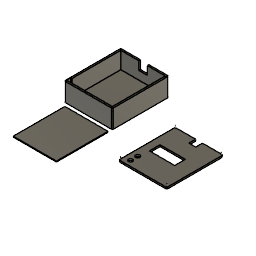
Case (Autodesk Fusion 360 design; units mm, degrees)
part number: 2025-12-30-11-50-45-676
Autodesk Fusion 360 part; units mm, degrees
sketch "Sketch1" plane through (0, 0, 0) normal (0, 0, 1) x (1, 0, 0)
  line L0 (0, 0) -> (53, 0)
  line L1 (53, 0) -> (53, -63)
  line L2 (53, -63) -> (0, -63)
  line L3 (0, -63) -> (0, 0)
  line L4 (-2, 2) -> (55, 2)
  line L5 (55, 2) -> (55, -65)
  line L6 (55, -65) -> (-2, -65)
  line L7 (-2, -65) -> (-2, 2)
  line L8 (0, -63) -> (-1.5, -63)
  line L9 (-1.5, -63) -> (-1.5, -58)
  line L10 (-1.5, -58) -> (0, -58)
  line L11 (0, -58) -> (0, -63)
  dimension "d1" = 53
  dimension "d2" = 63
  dimension "d7" = 1.5
  dimension "d8" = 5
  constraint horizontal L0
  constraint vertical L1
  constraint horizontal L2
  constraint vertical L3
  constraint coincident L0.start L3.end
  constraint horizontal L4
  constraint vertical L5
  constraint horizontal L6
  constraint vertical L7
  constraint horizontal L8
  constraint vertical L9
  constraint horizontal L10
  constraint vertical L11
  measures "d1" distance of L0.start L0.end
  measures "d2" distance of L0.start L2.end
  measures "d7" distance of L2.end L8.end
  measures "d8" distance of L2.end L10.end
extrude "Extrude1" add sketch "Sketch1" along normal blind 2 contours L0 L1 L2 L3 L11 | L3 L8 L9 L10 L11 makes body 1
extrude "Extrude2" add sketch "Sketch1" along normal blind 22 bodies 1
sketch "Sketch2" plane through (0, 0, 0) normal (0, 0, 1) x (1, 0, 0)
  line L0 (91.7333, -27) -> (148.7333, -27)
  line L1 (148.7333, -27) -> (148.7333, -94)
  line L2 (148.7333, -94) -> (91.7333, -94)
  line L3 (91.7333, -94) -> (91.7333, -27)
  line L4 (116.2333, -27) -> (124.2333, -27)
  line L5 (124.2333, -27) -> (124.2333, -35)
  line L6 (124.2333, -35) -> (116.2333, -35)
  line L7 (116.2333, -35) -> (116.2333, -27)
  line L8 (91.7333, -27) -> (116.2333, -27)
  line L9 (124.2333, -27) -> (148.7333, -27)
  line L10 (100.7333, -54) -> (130.7333, -54)
  line L11 (130.7333, -54) -> (130.7333, -66.5)
  line L12 (130.7333, -66.5) -> (100.7333, -66.5)
  line L13 (100.7333, -66.5) -> (100.7333, -54)
  circle A0 centre (99.2333, -87.5) radius 2.5
  circle A1 centre (99.2333, -79) radius 2.5
  dimension "d9" = 57
  dimension "d10" = 67
  dimension "d14" = 8
  dimension "d15" = 8
  dimension "d27" = 30
  dimension "d28" = 12.5
  dimension "d29" = 27
  dimension "d30" = 9
  dimension "d31" = 5
  dimension "d32" = 7.5
  dimension "d33" = 6.5
  dimension "d34" = 5
  dimension "d35" = 8.5
  constraint horizontal L0
  constraint vertical L1
  constraint horizontal L2
  constraint vertical L3
  constraint horizontal L4
  constraint vertical L5
  constraint horizontal L6
  constraint vertical L7
  constraint coincident L0 L4.start
  constraint equal L8 L9
  constraint horizontal L10
  constraint vertical L11
  constraint horizontal L12
  constraint vertical L13
  measures "d9" distance of L0.start L0.end
  measures "d10" distance of L0.start L2.end
  measures "d14" distance of L4.start L4.end
  measures "d15" distance of L4.start L6.end
  measures "d27" distance of L10.start L10.end
  measures "d28" distance of L10.start L12.end
  measures "d29" distance of L0 L10.start
  measures "d30" distance of L3 L13
  measures "d31" diameter of A0
  measures "d32" distance of L3 A0.centre
  measures "d33" distance of L2 A0.centre
  measures "d34" diameter of A1
  measures "d35" distance of A0.centre A1.centre
sketch "Sketch3" plane through (0, 0, 22) normal (0, 0, 1) x (-1, 0, 0)
  line L0 (1.5, 63) -> (1.5, 58)
  line L1 (1.5, 58) -> (0, 58)
  line L2 (0, 58) -> (0, 0)
  line L3 (0, 0) -> (-53, 0)
  line L4 (-53, 0) -> (-53, 63)
  line L5 (-53, 63) -> (1.5, 63)
  line L6 (2, 65) -> (-55, 65)
  line L7 (-55, 65) -> (-55, -2)
  line L8 (-55, -2) -> (2, -2)
  line L9 (2, -2) -> (2, 65)
  line L10 (-21.5, -2) -> (-31.5, -2)
  line L11 (-31.5, -2) -> (-31.5, 0)
  line L12 (-31.5, 0) -> (-21.5, 0)
  line L13 (-21.5, 0) -> (-21.5, -2)
  line L14 (2, -2) -> (-21.5, -2)
  line L15 (-31.5, -2) -> (-55, -2)
  line L16 (-91.7333, 27) -> (-148.7333, 27)
  line L17 (-91.7333, 94) -> (-91.7333, 27)
  line L18 (-148.7333, 94) -> (-91.7333, 94)
  circle A0 centre (1, -1) radius 0.5
  circle A1 centre (-54, -1) radius 0.5
  circle A2 centre (-54, 64) radius 0.5
  circle A3 centre (1, 64) radius 0.5
  dimension "d11" = 10
  dimension "d38" = 1
  dimension "d39" = 1
  dimension "d40" = 1
  constraint horizontal L10
  constraint vertical L11
  constraint horizontal L12
  constraint vertical L13
  constraint coincident L8 L10.start
  constraint coincident L8.end L9.start
  constraint coincident L7.end L8.start
  constraint equal L14 L15
  measures "d11" distance of L10.start L10.end
  measures "d38" diameter of A1
  measures "d39" diameter of A2
  measures "d40" diameter of A3
extrude "Extrude3" cut sketch "Sketch3" against normal blind 10 contours L3 L8 L10 L11 L12 L13 bodies 1
extrude "Extrude4" add sketch "Sketch2" along normal blind 2 separate body contours L0 L1 L2 L3 L5 L6 L7 L8 L9 makes body 2
extrude "Extrude5" cut sketch "Sketch3" against normal blind 3 contours A0 | A1 | A2 | A3 bodies 1
sketch "Sketch4" plane through (0, 0, 2) normal (0, 0, 1) x (-1, 0, 0)
  circle A0 centre (-99.2333, 79) radius 2.5
  circle A1 centre (-99.2333, 87.5) radius 2.5
  line L0 (-130.7333, 66.5) -> (-100.7333, 66.5)
  line L1 (-100.7333, 66.5) -> (-100.7333, 54)
  line L2 (-100.7333, 54) -> (-130.7333, 54)
  line L3 (-130.7333, 54) -> (-130.7333, 66.5)
  line L4 (-124.2333, 35) -> (-116.2333, 35)
  line L5 (-116.2333, 35) -> (-116.2333, 27)
  line L6 (-116.2333, 27) -> (-91.7333, 27)
  line L7 (-91.7333, 27) -> (-91.7333, 94)
  line L8 (-91.7333, 94) -> (-148.7333, 94)
  line L9 (-148.7333, 94) -> (-148.7333, 27)
  line L10 (-148.7333, 27) -> (-124.2333, 27)
  line L11 (-124.2333, 27) -> (-124.2333, 35)
  circle A2 centre (-92.7333, 28) radius 0.375
  circle A3 centre (-147.7333, 28) radius 0.375
  circle A4 centre (-92.7333, 93) radius 0.375
  circle A5 centre (-147.7333, 93) radius 0.375
  dimension "d43" = 0.75
  dimension "d44" = 1
  dimension "d45" = 1
  dimension "d46" = 0.75
  dimension "d47" = 1
  dimension "d48" = 1
  dimension "d49" = 0.75
  dimension "d50" = 1
  dimension "d51" = 1
  dimension "d52" = 0.75
  dimension "d53" = 1
  dimension "d54" = 1
  measures "d43" diameter of A2
  measures "d44" distance of L6 A2.centre
  measures "d45" distance of L7 A2.centre
  measures "d46" diameter of A3
  measures "d47" distance of L10 A3.centre
  measures "d48" distance of L9 A3.centre
  measures "d49" diameter of A4
  measures "d50" distance of L8 A4.centre
  measures "d51" distance of L7 A4.centre
  measures "d52" diameter of A5
  measures "d53" distance of L9 A5.centre
  measures "d54" distance of L8 A5.centre
extrude "Extrude6" add sketch "Sketch4" along normal blind 3 contours A2 | A3 | A4 | A5 bodies 2
sketch "Sketch5" plane through (0, 0, 0) normal (0, 0, 1) x (1, 0, 0)
  line L0 (55, -70) -> (3.5, -70)
  line L1 (3.5, -70) -> (3.5, -131.5)
  line L2 (3.5, -131.5) -> (55, -131.5)
  line L3 (55, -131.5) -> (55, -70)
  dimension "d57" = 51.5
  dimension "d58" = 61.5
  constraint horizontal L0
  constraint vertical L1
  constraint horizontal L2
  constraint vertical L3
  measures "d57" distance of L0.start L0.end
  measures "d58" distance of L0.start L2.end
extrude "Extrude7" add sketch "Sketch5" along normal blind 1 separate body makes body 3
fillet "Fillet1" radius 1 4 edges at (55, -65, 11) (-2, -65, 11) (-2, 2, 11) (55, 2, 11) on bodies 1
fillet "Fillet2" radius 1 4 edges at (91.7333, -94, 1) (148.7333, -94, 1) (148.7333, -27, 1) (91.7333, -27, 1) on bodies 2
